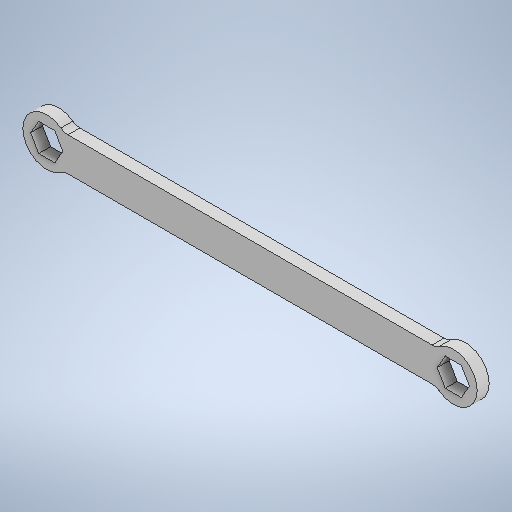
# Autodesk Inventor part: 2P.03.01.17.ZW.AileronCoupler
Saved by Autodesk Inventor 2025.2 (Build 292293000, 293)
## iProperties
Created: 2025-01-14
Part Number: 2P.03.01.17.ZW.AileronCoupler
Material: Generic
Document SubType Name: Modeling
Designer: Imist
Density: 1 g/cm^3
Appearance: Default
Author: Imist
Autodesk Inventor part; units mm, degrees
ref_plane "YZ Plane" through (0, 0, 0) normal (1, 0, 0) x (0, 1, 0)
ref_plane "XZ Plane" through (0, 0, 0) normal (0, 1, 0) x (-1, 0, 0)
ref_plane "XY Plane" through (0, 0, 0) normal (0, 0, 1) x (1, 0, 0)
sketch "Sketch1" plane through (0, 0, 0) normal (0, 0, 1) x (1, 0, 0)
  circle A0 centre (-51.129, 0.0665) radius 3.5
  circle A1 centre (50.996, 0.0665) radius 3.5
  arc A2 (-51.129, 6.0665) -> (-51.129, -5.9335) centre (-51.129, 0.0665) ccw
  arc A3 (50.996, -5.9335) -> (50.996, 6.0665) centre (50.996, 0.0665) ccw
  arc A4 (-51.129, -5.9335) -> (-47.5672, -4.7619) centre (-51.129, 0.0665) ccw
  line L0 (-51.129, 0.0665) -> (-46.8864, -4.1761) construction
  line L1 (-51.129, 0.0665) -> (-51.129, -5.9335) construction
  arc A5 (-47.5672, 4.895) -> (-51.129, 6.0665) centre (-51.129, 0.0665) ccw
  line L2 (-51.129, 0.0665) -> (-46.8864, 4.3092) construction
  line L3 (-51.129, 0.0665) -> (-51.129, 6.0665) construction
  arc A6 (50.996, 6.0665) -> (47.4342, 4.895) centre (50.996, 0.0665) ccw
  line L4 (50.996, 0.0665) -> (46.7533, 4.3092) construction
  line L5 (50.996, 0.0665) -> (50.996, 6.0665) construction
  arc A7 (47.4342, -4.7619) -> (50.996, -5.9335) centre (50.996, 0.0665) ccw
  line L6 (50.996, 0.0665) -> (46.7533, -4.1761) construction
  line L7 (50.996, 0.0665) -> (50.996, -5.9335) construction
  line L8 (-45.7864, 4.3092) -> (45.6533, 4.3092)
  line L9 (-45.7864, -4.1761) -> (45.6533, -4.1761)
  arc A8 (-47.5672, 4.895) -> (-45.7864, 4.3092) centre (-45.7864, 7.3092) ccw
  arc A9 (-45.7864, -4.1761) -> (-47.5672, -4.7619) centre (-45.7864, -7.1761) ccw
  arc A10 (45.6533, 4.3092) -> (47.4342, 4.895) centre (45.6533, 7.3092) ccw
  arc A11 (47.4342, -4.7619) -> (45.6533, -4.1761) centre (45.6533, -7.1761) ccw
  line L10 (-47.0876, 0.0665) -> (-49.1083, -3.4335)
  line L11 (-49.1083, -3.4335) -> (-53.1498, -3.4335)
  line L12 (-53.1498, -3.4335) -> (-55.1705, 0.0665)
  line L13 (-55.1705, 0.0665) -> (-53.1498, 3.5665)
  line L14 (-53.1498, 3.5665) -> (-49.1083, 3.5665)
  line L15 (-49.1083, 3.5665) -> (-47.0876, 0.0665)
  line L16 (55.0374, 0.0665) -> (53.0167, -3.4335)
  line L17 (53.0167, -3.4335) -> (48.9752, -3.4335)
  line L18 (48.9752, -3.4335) -> (46.9545, 0.0665)
  line L19 (46.9545, 0.0665) -> (48.9752, 3.5665)
  line L20 (48.9752, 3.5665) -> (53.0167, 3.5665)
  line L21 (53.0167, 3.5665) -> (55.0374, 0.0665)
  point P0 (0, 0)
  point P1 (46.7533, 4.3092)
  dimension "d0" = 7
  dimension "d1" = 7
  dimension "d2" = 102.125
  dimension "d3" = 6
  dimension "d4" = 6
  dimension "d5" = 45
  dimension "d6" = 45
  dimension "d7" = 45
  dimension "d8" = 45
  dimension "d9" = 3
  constraints: 44 end point, 24 point on circle, 12 centre point, 10 tangent, 9 coincident, 4 point on line, 3 equal radius, 1 horizontal, 26 other
  measures "d0" diameter of A0
  measures "d1" diameter of A1
  measures "d2" distance of L1.end L7.end
  measures "d3" radius of A2
  measures "d4" radius of A3
  measures "d5" angle of L1 L0
  measures "d6" angle of L2 L3
  measures "d7" angle of L5 L4
  measures "d8" angle of L6 L7
  measures "d9" radius of A8
extrude "Extrusion2" add sketch "Sketch1" along normal blind 3
body "Solid2"
